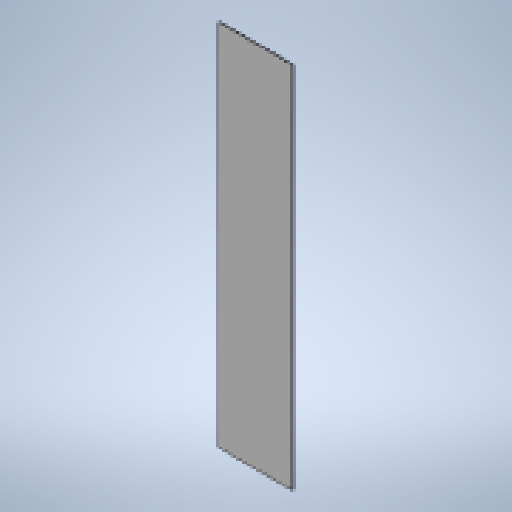
# Autodesk Inventor part: Ограждающий борт
Saved by Autodesk Inventor 2025 (Build 290162010, 162A)
## iProperties
Created: 2025-01-20
Part Number: Ограждающий борт
Material: Stainless Steel
Document SubType Name: Sheet Metal
Designer: pokla
Density: 8 g/cm^3
Sheet Metal Rule: AISI304 2mm Die16
Appearance: Default
Author: pokla
Autodesk Inventor part; units mm, degrees
ref_plane "YZ Plane" through (0, 0, 0) normal (1, 0, 0) x (0, 1, 0)
ref_plane "XZ Plane" through (0, 0, 0) normal (0, 1, 0) x (-1, 0, 0)
ref_plane "XY Plane" through (0, 0, 0) normal (0, 0, 1) x (1, 0, 0)
sketch "Sketch1" plane through (0, 0, 0) normal (0, 1, 0) x (-1, 0, 0)
  line L0 (100, 625) -> (-100, 625)
  line L1 (-100, 625) -> (-100, -625)
  line L2 (-100, -625) -> (100, -625)
  line L3 (100, -625) -> (100, 625)
  line L4 (100, 625) -> (-100, -625) construction
  point P0 (0, 0)
  point P1 (0, 0)
  dimension "d0" = 200
  dimension "d1" = 1250
  measures "d0" distance of L0.start L0.end
  measures "d1" distance of L2.end L0.start
extrude "Plate1" add sketch "Sketch1" along normal blind 2
equation "\"d2\" = Thickness"
equation "\"BendReliefWidth\" = Thickness"
equation "\"BendReliefDepth\" = 0.5 * Thickness"
equation "\"CornerReliefSize\" = 4 * Thickness"
equation "\"MinimumRemnant\" = 2 * Thickness"
equation "\"TransitionRadius\" = BendRadius"
equation "\"JacobiRadiusSize\" = BendRadius"
equation "\"GapSize\" = Thickness"
equation "\"Thickness\" = 2"
equation "\"BendRadius\" = 2.75"
body "Solid1"
